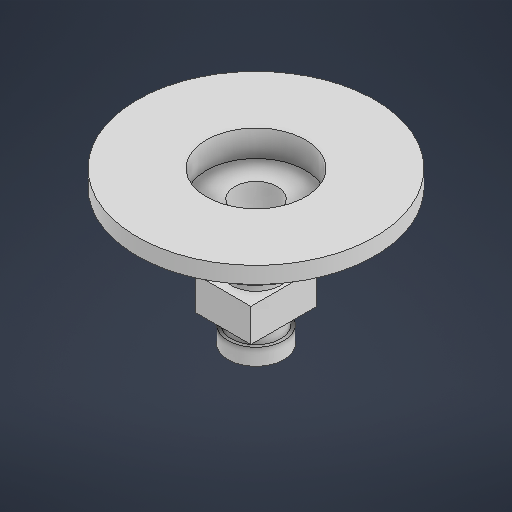
# Autodesk Inventor part: Axis1_bottom
Saved by Autodesk Inventor 2026.1 (Build 301233020, 233B)
## iProperties
Created: 2025-10-29
Part Number: Axis1_bottom
Material: Generic
Document SubType Name: Modeling
Designer: Piter
Density: 1 g/cm^3
Appearance: Default
Author: Piter
Autodesk Inventor part; units mm, degrees
ref_plane "YZ Plane" through (0, 0, 0) normal (1, 0, 0) x (0, 1, 0)
ref_plane "XZ Plane" through (0, 0, 0) normal (0, 1, 0) x (-1, 0, 0)
ref_plane "XY Plane" through (0, 0, 0) normal (0, 0, 1) x (1, 0, 0)
sketch "Sketch1" plane through (0, 0, 0) normal (0, 1, 0) x (-1, 0, 0)
  circle A0 centre (0, 0) radius 36
  circle A1 centre (0, 0) radius 15
  dimension "d0" = 72
  dimension "d1" = 30
  constraints: 2 centre point, 2 coincident
  measures "d0" diameter of A0
  measures "d1" diameter of A1
extrude "Extrusion1" add sketch "Sketch1" along normal blind 5
sketch "Sketch2" plane through (0, 0, 0) normal (0, -1, 0) x (1, 0, 0)
  circle A0 centre (0, 0) radius 36 projected
  circle A1 centre (0, 0) radius 15 projected
  circle A2 centre (0, 0) radius 20.05
  dimension "d4" = 40.1
  constraints: 1 centre point, 1 coincident
  measures "d4" diameter of A2
extrude "Extrusion2" add sketch "Sketch2" along normal blind 11.5 contours A2
sketch "Sketch3" plane through (0, -11.5, 0) normal (0, -1, 0) x (1, 0, 0)
  circle A0 centre (0, 0) radius 7.5
  circle A1 centre (0, 0) radius 20.05 projected
  circle A2 centre (0, 0) radius 15 projected
  circle A3 centre (0, 0) radius 6.5
  dimension "d7" = 15
  dimension "d8" = 13
  constraints: 2 centre point, 2 coincident
  measures "d7" diameter of A0
  measures "d8" diameter of A3
extrude "Extrusion3" add sketch "Sketch3" along normal blind 29.5 and the other way blind 8.5 contours A0
extrude "Extrusion4" add sketch "Sketch3" against normal up to surface (8.5 mm away) contours A2
sketch "Sketch4" plane through (0, -41, 0) normal (0, -1, 0) x (1, 0, 0)
  circle A0 centre (0, 0) radius 7.5 projected
  circle A1 centre (0, 0) radius 6.5 projected
  circle A2 centre (0, 0) radius 8.45
  dimension "d15" = 16.9
  constraints: 1 centre point, 1 coincident
  measures "d15" diameter of A2
extrude "Extrusion5" add sketch "Sketch4" against normal blind 5 contours A2
sketch "Sketch5" plane through (0, -36, 0) normal (0, 1, 0) x (1, 0, 0)
  point P0 (0, 0)
sketch "Sketch6" plane through (0, 0, 0) normal (0, 0, 1) x (1, 0, 0)
  line L0 (8.45, -36) -> (-8.45, -36) projected
  line L1 (-8.45, -41) -> (8.45, -41) projected
  line L2 (8.45, -32) -> (-8.45, -32)
  line L3 (-8.45, -32) -> (-8.45, -22)
  line L4 (-8.45, -22) -> (8.45, -22)
  line L5 (8.45, -22) -> (8.45, -32)
  point P0 (0, 0)
  dimension "d18" = 10
  dimension "d21" = 9
  constraints: 8 end point, 2 parallel, 1 horizontal, 1 perpendicular
  measures "d18" distance of L2.end L3.end
  measures "d21" distance between parallel lines of L1 L2
extrude "Extrusion6" add sketch "Sketch6" along normal mid plane 20
body "Solid1"
